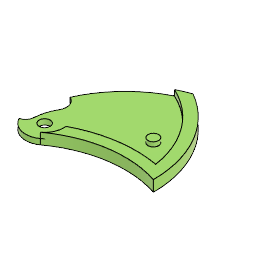
Leaf (Autodesk Fusion 360 design; units mm, degrees)
part number: 2026-06-05-20-37-06-533
Autodesk Fusion 360 part; units mm, degrees
note: some values were not read from the file. Chosen so that the rebuilt part matches the saved one: a direction; which face or edge a step refers to. Set by a fixed rule: which sketch regions a step uses.
sketch "Sketch1" plane through (0, 0, 0) normal (0, 0, 1) x (1, 0, 0)
  circle A0 centre (0, 0) radius 49.2 construction
  circle A1 centre (-49.2, 0) radius 2.5
  line L0 (0, 0) -> (-15.2036, -46.792) construction
  line L1 (0, 0) -> (44.5, 0) construction
  circle A2 centre (-49.2, 0) radius 8.6381
  arc A3 (-24.6, 42.6084) -> (-57.7848, 0.9582) centre (-8.0933, -4.5883) ccw
  line L2 (-49.2, 0) -> (0, 0) construction
  arc A4 (0, 0) -> (-24.6, 42.6084) centre (-49.2, 0) ccw
  arc A5 (0, 0) -> (-44.1227, -6.9883) centre (-15.2036, -46.792) ccw
  arc A6 (-5.485, 6.5296) -> (-30.5627, 40.0786) centre (-49.2, 0) ccw
  arc A7 (-5.485, 6.5296) -> (-40.629, 1.0744) centre (-15.2036, -46.792) ccw
  line L3 (0, 0) -> (-16.9706, 16.9706) construction
  circle A8 centre (-16.9706, 16.9706) radius 2.4
  dimension "d1" = 98.4
  dimension "d2" = 5
  dimension "d5" = 50
  dimension "d9" = 72
  dimension "d12" = 4.8
  dimension "d13" = 5
  dimension "d14" = 5
  dimension "d15" = 24
  dimension "d20" = 45
  constraint coincident A0.centre L0.start
  constraint coincident A0 A1.centre
  constraint concentric A1 A4
  constraint horizontal L1
  constraint coincident A0 L0.end
  constraint concentric A1 A2
  constraint coincident A0 A3.start
  constraint coincident A2 A3.end
  constraint tangent A2 A3
  constraint horizontal A0.centre A1.centre
  constraint coincident A1.centre A2.centre
  constraint coincident L0 A0.centre
  constraint coincident A0.centre A5
  constraint tangent A2 A5
  constraint coincident L0.end A5.centre
  constraint coincident A2 A5.end
  constraint coincident A2 A7.end
  constraint coincident A3 A6.end
  constraint coincident L3.end A8.centre
  measures "d1" diameter of A0
  measures "d2" diameter of A1
  measures "d5" radius of A3
  measures "d9" angle of L0 L2
  measures "d12" diameter of A8
  measures "d13" distance of A4 A6
  measures "d14" distance of A5 A7
  measures "d15" distance of A0.centre L3.end
  measures "d20" angle of L2 L3
extrude "Extrude1" add sketch "Sketch1" along normal blind 2.5 contours A2 | A2 A3 A4 A5 A6 A7 | A2 A3 A6 A7 | A8
extrude "Extrude2" add sketch "Sketch1" along normal blind 5 contours A2 A3 A4 A5 A6 A7
extrude "Extrude3" add sketch "Sketch1" along normal blind 4.5 contours A8
sketch "Sketch2" plane through (0, 0, 2.5) normal (0, 0, 1) x (-1, 0, 0)
  circle A0 centre (16.9706, -16.9706) radius 2.4
  arc A1 (44.1227, 6.9883) -> (40.629, -1.0744) centre (49.2, 0) ccw
  arc A2 (5.485, -6.5296) -> (40.629, -1.0744) centre (15.2036, 46.792) ccw
  arc A3 (5.485, -6.5296) -> (30.5627, -40.0786) centre (49.2, 0) ccw
  arc A4 (30.5627, -40.0786) -> (57.7848, -0.9582) centre (8.0933, 4.5883) ccw
  arc A5 (57.7848, -0.9582) -> (44.1227, 6.9883) centre (49.2, 0) ccw
  circle A6 centre (49.2, 0) radius 2.5
  circle A7 centre (57.8824, 0) radius 4
  circle A8 centre (55.5172, -11.2541) radius 5
  arc A9 (51.1977, -8.7358) -> (53.8886, 0.2229) centre (33.9197, 1.3375) ccw
  line L0 (61.8536, -0.4792) -> (60.4812, -11.8531)
  dimension "d21" = 8
  dimension "d22" = 10
  dimension "d23" = 11.5
  dimension "d24" = 20
  constraint coincident A4 A7.centre
  constraint coincident A4 A8.centre
  constraint coincident A7 A9.end
  constraint tangent A7 A9
  constraint coincident A8 A9.start
  constraint tangent A8 A9
  constraint coincident A7 L0.start
  constraint coincident A8 L0.end
  constraint tangent A8 L0
  constraint horizontal A1.centre A7.centre
  constraint tangent A7 L0
  measures "d21" diameter of A7
  measures "d22" diameter of A8
  measures "d23" distance of A7.centre A8.centre
  measures "d24" radius of A9
extrude "Extrude4" cut sketch "Sketch2" against normal through all contours A4 A5 A7 | A4 A5 A7 | A4 A7 A8 A9 | A4 A8 | A4 A8
